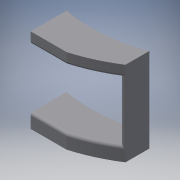
# Autodesk Inventor part: Stiff_motor
Saved by Autodesk Inventor 2019.3 (Build 233278000, 278)
## iProperties
Created: 2020-09-24
Part Number: Stiff_motor
Material: Generisch
Document SubType Name: Modeling
Designer: Nicolas Frick
Density: 1 g/cm^3
Appearance: Vorgabe
Author: Nicolas Frick
Autodesk Inventor part; units mm, degrees
ref_plane "YZ Plane" through (0, 0, 0) normal (1, 0, 0) x (0, 1, 0)
ref_plane "XZ Plane" through (0, 0, 0) normal (0, 1, 0) x (-1, 0, 0)
ref_plane "XY Plane" through (0, 0, 0) normal (0, 0, 1) x (1, 0, 0)
sketch "Skizze1" plane through (0, 0, 0) normal (0, 0, 1) x (1, 0, 0)
  line L0 (9, 36) -> (9, 6) construction
  line L1 (-9, 36) -> (9, 36) construction
  line L2 (-9, 6) -> (-9, 36) construction
  line L3 (-9, 6) -> (9, 6) construction
  line L4 (9, 36) -> (9, 6) construction
  line L5 (-9, 42) -> (9, 42) construction
  line L6 (9, 6) -> (9, 0) construction
  line L7 (-9, 42) -> (-31, 42) construction
  line L8 (2.1623, -5) -> (-7.3221, -5) construction
  line L9 (-9, 0) -> (9, 0) construction
  line L10 (2.1623, 6.8548) -> (2.1623, -5) construction
  line L11 (4.0374, -5) -> (4.0374, 6.8548) construction
  line L12 (4.0374, -5) -> (2.1623, -5) construction
  line L13 (9, 42) -> (9, 36) construction
  line L14 (32.5442, 50) -> (-21.2, 50) construction
  line L15 (-22.4813, -15) -> (-22.4813, 53) construction
  arc A0 (-22.4813, 53) -> (-24.4813, 55) centre (-24.4813, 53) ccw construction
  arc A1 (-24.6813, -15) -> (-22.6813, -13) centre (-24.6813, -13) ccw construction
  line L16 (-22.6813, -13) -> (-22.6813, -12) construction
  line L17 (-24.4813, -13) -> (-47, -13) construction
  line L18 (-24.4813, 53) -> (-24.4813, -13) construction
  line L19 (-47, 53) -> (-24.4813, 53) construction
  line L20 (-47, -13) -> (-47, 53) construction
  line L21 (-9, 6) -> (-9, 0) construction
  line L22 (-8.7, -6) -> (-8.7, -4) construction
  line L23 (-8.7, -6) -> (-8.7, -4) construction
  line L24 (-8.7, -4) -> (-7.7, -4) construction
  line L25 (-7.7, -4) -> (-7.7, -6) construction
  line L26 (-7.7, -6) -> (-4.7, -6) construction
  line L27 (-4.7, 1) -> (-4.7, -6) construction
  line L28 (-4.7, 1) -> (-9.7, 1) construction
  line L29 (-9.7, 1) -> (-9.7, -6) construction
  line L30 (-9.7, -6) -> (-8.7, -6) construction
  line L31 (-9, 0.5858) -> (-9, 7.4142) construction
  line L32 (-31, 0) -> (-9, 0) construction
  line L33 (-21.2, 52) -> (-21.2, 50) construction
  line L34 (-21.2, -10) -> (32.5442, -10) construction
  line L35 (-21.2, -10) -> (-21.2, -12) construction
  line L36 (32.2, 50) -> (32.2, 35.4011) construction
  line L37 (32.2, 4.5989) -> (32.2, -10) construction
  line L38 (-21.9813, -10) -> (32.2, -10)
  line L39 (32.2, -10) -> (32.2, 50)
  line L40 (32.2, 50) -> (-21.9813, 50)
  line L41 (-21.9813, 42) -> (29.0187, 42)
  line L42 (29.0187, 42) -> (29.0187, 0)
  line L43 (29.0187, 0) -> (-21.9813, 0)
  line L44 (-21.9813, -10) -> (-21.9813, 0)
  line L45 (-21.9813, 42) -> (-21.9813, 50)
  point P0 (0, 0)
  constraints: 16 end point, 4 perpendicular, 2 horizontal, 2 parallel, 2 point on line
extrude "Extrusion1" add sketch "Skizze1" along normal mid plane 30
sketch "Skizze2" plane through (-21.9813, 50, 15) normal (0, 1, 0) x (1, 0, 0)
  circle A0 centre (33.5439, 8.6575) radius 2.15 construction
  circle A1 centre (12.1205, 3.0946) radius 2.15 construction
  arc A2 (-10.3687, -0.3954) -> (-6.0687, -0.3954) centre (-8.2187, -0.3954) ccw construction
  line L0 (-10.3687, -0.3954) -> (-10.3687, 4.6046) construction
  arc A3 (-6.0687, 4.6046) -> (-10.3687, 4.6046) centre (-8.2187, 4.6046) ccw construction
  line L1 (-6.0687, 4.6046) -> (-6.0687, -0.3954) construction
  line L2 (-6.0687, 21.1993) -> (-6.0687, 16.1993) construction
  arc A4 (-10.3687, 16.1993) -> (-6.0687, 16.1993) centre (-8.2187, 16.1993) ccw construction
  line L3 (-10.3687, 16.1993) -> (-10.3687, 21.1993) construction
  arc A5 (-6.0687, 21.1993) -> (-10.3687, 21.1993) centre (-8.2187, 21.1993) ccw construction
  line L4 (58.3, 29.6207) -> (63.3, 29.6207) construction
  line L5 (58.3, 29.6207) -> (58.3, 23.282) construction
  line L6 (58.3, 23.282) -> (57.1813, 23.282) construction
  line L7 (57.1813, 23.282) -> (57.1813, 29.0056) construction
  arc A6 (-9.2981, 25.6207) -> (57.1813, 29.0056) centre (18.9366, 125.6108) ccw construction
  line L8 (-18.2187, 25.6207) -> (-9.2981, 25.6207) construction
  line L9 (-18.2187, -4.3793) -> (-18.2187, 25.6207) construction
  line L10 (-2.7, -4.3793) -> (-18.2187, -4.3793) construction
  arc A7 (-0.7916, -2.3814) -> (-2.7, -4.3793) centre (-0.7, -4.3793) ccw construction
  arc A8 (-0.7916, -2.3814) -> (63.3, 22.1907) centre (-5.7872, 106.5198) ccw construction
  line L11 (63.3, 29.6207) -> (63.3, 22.1907) construction
  arc A9 (-0.7, -4.3793) -> (62.5308, 19.0147) centre (-5.7872, 106.5198) ccw construction
  arc A10 (-0.7, 25.6207) -> (57.1813, 31.16) centre (18.9366, 125.6108) ccw construction
  arc A11 (-0.7, 25.6207) -> (57.1813, 31.16) centre (18.9366, 125.6108) ccw construction
  line L12 (51, 0) -> (0, 0) construction
  line L13 (54.1813, 0) -> (54.1813, 30) construction
  arc A12 (25.5, 0) -> (54.1813, 13.0946) centre (-5.8671, 106.662) ccw
  line L14 (0, 0) -> (0, 30) construction
  arc A13 (0, 25.4858) -> (54.1813, 30) centre (18.9366, 125.6108) ccw
  line L15 (54.1813, 0) -> (25.5, 0)
  line L16 (54.1813, 13.0946) -> (54.1813, 0)
  line L17 (0, 25.9057) -> (0, 30)
  line L18 (0, 30) -> (51, 30) projected
  line L19 (0, 30) -> (54.1813, 30)
  line L20 (0, 25.9057) -> (0, 25.4858)
  point P0 (21.9813, 15)
  constraints: 10 end point, 7 point on circle, 5 collinear, 3 point on line, 2 centre point, 1 concentric, 1 midpoint
extrude "Extrusion2" cut sketch "Skizze2" against normal through all
fillet "Rundung1" radius 2 5 edges at (16.6181, 0, 10.237) (-9.2313, 0, 15) (-9.2313, 42, 15) (16.6181, 42, 10.237) (29.0187, 21, 3.8723)
